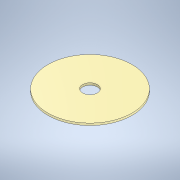
# Autodesk Inventor part: Прокладка
Saved by Autodesk Inventor 2022 (Build 260153000, 153)
## iProperties
Created: 2024-04-28
Part Number: Прокладка
Material: Типовые
Document SubType Name: Modeling
Designer: Pavel
Density: 1 g/cm^3
Appearance: По умолчанию
Author: Pavel
Autodesk Inventor part; units mm, degrees
ref_plane "YZ Plane" through (0, 0, 0) normal (1, 0, 0) x (0, 1, 0)
ref_plane "XZ Plane" through (0, 0, 0) normal (0, 1, 0) x (-1, 0, 0)
ref_plane "XY Plane" through (0, 0, 0) normal (0, 0, 1) x (1, 0, 0)
sketch "Эскиз1" plane through (0, 0, 0) normal (0, 1, 0) x (-1, 0, 0)
  circle A0 centre (0, 0) radius 10
  circle A1 centre (0, 0) radius 1.75
  dimension "d0" = 20
  dimension "d1" = 3.5
  constraints: 2 centre point, 2 coincident
  measures "d0" diameter of A0
  measures "d1" diameter of A1
extrude "Выдавливание1" add sketch "Эскиз1" along normal blind 0.5
